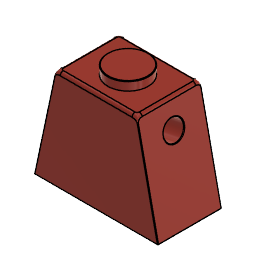
LegoFigureFinal (Autodesk Fusion 360 archive; units mm, degrees)
design "Torso"
part number: 2026-05-19-12-12-37-502
Autodesk Fusion 360 part; units mm, degrees
sketch "Body" plane through (0, 0, 0) normal (0, 1, 0) x (1, 0, 0)
  line L0 (0, 0) -> (0, -12.7) construction
  line L1 (-5.08, -12.7) -> (5.08, -12.7)
  line L2 (-7.7795, 0) -> (7.7795, 0)
  line L3 (-5.08, -12.7) -> (-7.7795, 0)
  line L4 (5.08, -12.7) -> (7.7795, 0)
  dimension "d1" = 12.7
  dimension "d2" = 10.16
  dimension "d3" = 78
  constraint coincident L0.start origin
  constraint vertical L0
  constraint perpendicular L0 L1
  constraint coincident L0.end L1
  constraint symmetric L0 L1.start L1.end
  constraint horizontal L2
  constraint coincident L0.start L2
  constraint symmetric L0 L2.start L2.end
  measures "d1" distance of L0.start L0.end
  measures "d2" distance of L1.start L1.end
  measures "d3" angle of L2 L3
extrude "Extrude1" add sketch "Body" along normal mid plane 8.001
sketch "Neck" plane through (0, 0, 12.7) normal (0, 0, 1) x (-1, 0, 0)
  line L0 (-5.08, 4.0005) -> (-5.08, -4.0005)
  line L1 (-5.08, -4.0005) -> (5.08, -4.0005)
  line L2 (5.08, -4.0005) -> (5.08, 4.0005)
  line L3 (5.08, 4.0005) -> (-5.08, 4.0005)
  circle A0 centre (0, 0) radius 2.54
  dimension "d6" = 5.08
  constraint coincident A0.centre origin
  measures "d6" diameter of A0
extrude "Extrude2" add sketch "Neck" along normal blind 1.095 contours A0
sketch "LegHoles" plane through (0, 0, 0) normal (0, 0, -1) x (1, 0, 0)
  line L0 (-7.7795, 4.0005) -> (-7.7795, -4.0005)
  line L1 (-7.7795, -4.0005) -> (7.7795, -4.0005)
  line L2 (7.7795, -4.0005) -> (7.7795, 4.0005)
  line L3 (7.7795, 4.0005) -> (-7.7795, 4.0005)
  circle A0 centre (3.81, 0) radius 2.54
  circle A1 centre (-3.81, 0) radius 2.54
  dimension "d10" = 5.08
  dimension "d11" = 5.08
  dimension "d12" = 3.81
  dimension "d13" = 3.81
  constraint horizontal origin A1.centre
  constraint horizontal origin A0.centre
  measures "d10" diameter of A0
  measures "d11" diameter of A1
  measures "d12" distance of origin A1.centre
  measures "d13" distance of origin A0.centre
extrude "Extrude3" cut sketch "LegHoles" against normal blind 5.08 contours A0 | A1
sketch "HelperLine" plane through (0, -4.0005, 0) normal (0, -1, 0) x (1, 0, 0)
  line L0 (5.08, 12.7) -> (-5.08, 12.7)
  line L1 (-5.08, 12.7) -> (-7.7795, 0)
  line L2 (-7.7795, 0) -> (7.7795, 0)
  line L3 (7.7795, 0) -> (5.08, 12.7)
  line L4 (-5.7549, 9.525) -> (5.7549, 9.525)
  dimension "d16" = 9.525
  constraint coincident L1 L4.start
  constraint coincident L3 L4.end
  constraint horizontal L4
  measures "d16" distance of L2 L4
sketch "ArmHoles" plane through (7.4432, 0, 1.5821) normal (0.978148, 0, 0.207912) x (0, 1, 0)
  line L0 (-4.0005, -1.6174) -> (4.0005, -1.6174)
  line L1 (4.0005, -1.6174) -> (4.0005, 11.3663)
  line L2 (4.0005, 11.3663) -> (-4.0005, 11.3663)
  line L3 (-4.0005, 11.3663) -> (-4.0005, -1.6174)
  line L4 (-4.0005, 10.5134) -> (-4.0005, 8.1204)
  line L5 (-4.0005, 8.1204) -> (0, 8.1204)
  constraint coincident L4.end L5.start
  constraint perpendicular L3 L5
  constraint vertical origin L5.end
hole "Hole1" at (5.7549, 0, 9.525) direction (-0.978148, 0, -0.207912) diameter 2.54 depth 5.08 tip angle 118
mirror "Mirror1" about plane through (0, 0, 0) normal (1, 0, 0) of "Hole1"
fillet "Fillet1" radius 0.381 4 edges at (0, -4.0005, 12.7) (-5.08, 0, 12.7) (0, 4.0005, 12.7) (5.08, 0, 12.7)
fillet "Fillet1" radius 0.0635 7 edges at (6.4297, -4.0005, 6.35) (6.4297, 4.0005, 6.35) (-6.4297, -4.0005, 6.35) (-6.4297, 4.0005, 6.35) (2.3681, 0.9185, 13.795) (5.6594, -1.1841, 9.9742) (-5.8504, -1.1841, 9.0758) 1 faces at (-1.0816, 3.4924, 0)
equation "d13 = d12"
equation "d18 = ( 1.27 * 2 ) * 1 mm"
named bodies: "Torso"

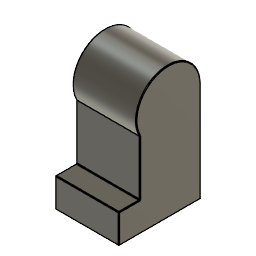
design "LeftLeg"
part number: 2026-05-19-14-25-58-594
Autodesk Fusion 360 part; units mm, degrees
sketch "LegOutline" plane through (0, 0, 0) normal (1, 0, 0) x (0, 1, 0)
  line L0 (3.5052, 0) -> (3.5052, -10.795)
  line L1 (3.5052, -10.795) -> (-5.3848, -10.795)
  line L2 (-5.3848, -10.795) -> (-5.3848, -7.62)
  line L3 (-3.0988, -1.6383) -> (-3.0988, -7.62)
  line L4 (-5.3848, -7.62) -> (-3.0988, -7.62)
  arc A0 (3.5052, 0) -> (-3.0988, -1.6383) centre (0, 0) ccw
  circle A1 centre (0, 0) radius 0.8255
  dimension "d1" = 7.0104
  dimension "d2" = 10.795
  dimension "d3" = 8.89
  dimension "d4" = 3.175
  dimension "d5" = 6.604
  dimension "d6" = 1.651
  constraint coincident A0.centre A1.centre
  constraint vertical L0
  constraint tangent L0 A0
  constraint perpendicular L0 L1
  constraint perpendicular L1 L2
  constraint vertical L3
  constraint perpendicular L3 L4
  constraint concentric A0 A1
  measures "d1" diameter of A0
  measures "d2" distance of L0.start L0.end
  measures "d3" distance of L0.end L1.end
  measures "d4" distance of L1.end L2.end
  measures "d5" distance of L0 L3
  measures "d6" diameter of A1
extrude "Extrude1" add sketch "LegOutline" against normal blind 6.9088 contours L0 L1 L2 L3 L4 A0 | A1
extrude "Extrude2" cut sketch "LegOutline" along normal blind 5.08 from surface at -6.9088 contours A1
fillet "Fillet1" radius 0.0635 2 edges at (-3.4544, -3.0988, -7.62) (-3.4544, -5.3848, -7.62) 3 faces at (-6.9088, 0.236, -6.3945) (0, 1.3039, -6.1383) (-4.6059, 0.5419, -10.795)
named bodies: "Leg"

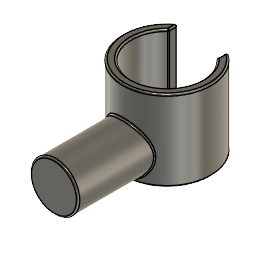
design "LeftHand"
part number: 2026-05-19-15-14-27-617
Autodesk Fusion 360 part; units mm, degrees
sketch "HandOutline" plane through (0, 0, 0) normal (0, 0, 1) x (1, 0, 0)
  circle A0 centre (0, 0) radius 1.7272
  circle A1 centre (0, 0) radius 1.397
  line L0 (-0.9525, 1.4408) -> (-0.9525, 1.0219)
  line L1 (0.9525, 1.4408) -> (0.9525, 1.0219)
  line L2 (0, 1.7272) -> (0, -1.7272) construction
  dimension "d1" = 3.4544
  dimension "d2" = 2.794
  dimension "d3" = 1.905
  constraint coincident A0.centre A1.centre
  constraint concentric A0 A1
  constraint coincident A0 L0.start
  constraint coincident A1 L0.end
  constraint vertical L0
  constraint coincident A0 L1.start
  constraint coincident A1 L1.end
  constraint parallel L0 L1
  constraint coincident A0 L2.start
  constraint coincident A0 L2.end
  constraint vertical L2
  constraint symmetric L0 L1 L2
  measures "d1" diameter of A0
  measures "d2" diameter of A1
  measures "d3" distance of L0 L1
extrude "Extrude1" add sketch "HandOutline" along normal blind 2.159 and the other way blind 1.016 contours A0 A1 L0 L1 picked at (-1.1455, 1.1363)
sketch "HandJoint" plane through (0, 0, 0) normal (0, 1, 0) x (1, 0, 0)
  circle A0 centre (0, 0) radius 0.9525
  dimension "d8" = 1.905
  constraint coincident A0.centre origin
  measures "d8" diameter of A0
extrude "Extrude2" add sketch "HandJoint" against normal blind 4.445
delete_face "DeleteFace1" 1 faces at (-0.0029, -0.4657, -0.9525)
fillet "Fillet1" radius 0.0635 2 edges at (-0.888, -4.445, -0.3444) (-0.9525, -1.4408, 0) 4 faces at (0, -1.6141, 2.159) (-0.9525, 1.3012, 0.0423) (0.9525, 1.3012, 0.0423) (0, -1.6141, -1.016)
named bodies: "Hand"
